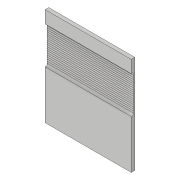
# Autodesk Inventor part: 00_chip_fibers_01
Saved by Autodesk Inventor 2019.4 (Build 234330000, 330)
## iProperties
Created: 2020-05-10
Part Number: 00_chip_fibers_01
Material: Generic
Document SubType Name: Modeling
Designer: diederichbenedict
Density: 1 g/cm^3
Appearance: Default
Author: diederichbenedict
Autodesk Inventor part; units mm, degrees
ref_plane "YZ Plane" through (0, 0, 0) normal (1, 0, 0) x (0, 1, 0)
ref_plane "XZ Plane" through (0, 0, 0) normal (0, 1, 0) x (-1, 0, 0)
ref_plane "XY Plane" through (0, 0, 0) normal (0, 0, 1) x (1, 0, 0)
sketch "Sketch1" plane through (0, 0, 0) normal (0, 0, 1) x (1, 0, 0)
  line L0 (0, 0) -> (23.76, 0)
  line L1 (23.76, 0) -> (23.76, 27)
  line L2 (23.76, 27) -> (0, 27)
  line L3 (0, 27) -> (0, 0)
  dimension "d0" = 23.76
  dimension "d1" = 27
  constraints: 8 end point, 2 parallel, 1 horizontal, 1 perpendicular
  measures "d0" distance of L2.end L1.end
  measures "d1" distance of L1.end L0.end
extrude "Extrusion1" add sketch "Sketch1" along normal blind 1
sketch "Sketch3" plane through (23.76, 0, 0) normal (1, 0, 0) x (0, 0, -1)
  line L0 (-1, 0) -> (-1, 27) projected
  line L1 (0, 0) -> (-1, 0) projected
  line L2 (0, 0) -> (0, 27) projected
  line L3 (0, 27) -> (-1, 27) projected
  circle A0 centre (-0.8098, 23.2257) radius 0.4098
  line L4 (-0.4, 23.7) -> (-0.4, 16.95) projected
  point P0 (0, 0)
  constraints: 1 centre point, 1 tangent
extrude "Extrusion3" cut sketch "Sketch3" against normal through all contours A0 L0 | L0 A0
pattern_linear "Rectangular Pattern2" count 20 spacing 0.5 along (0, -1, 0) of "Extrusion3"
body "Solid1"
